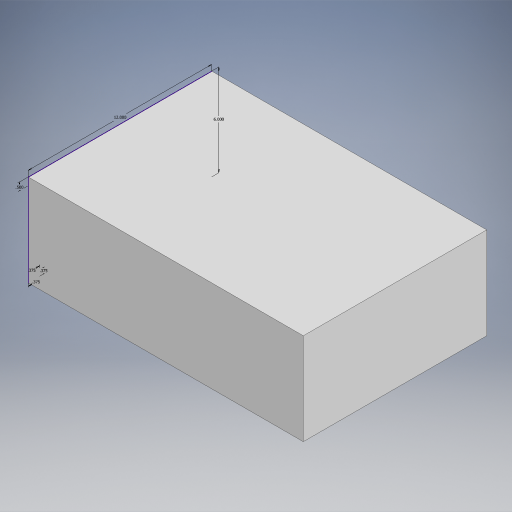
# Autodesk Inventor part: Typ_rect-01
Saved by Autodesk Inventor 2023 (Build 270158000, 158)
## iProperties
RuleStatus: InUse
Created: 2022-10-23
Part Number: Typ_rect-01
Material: Generic
Document SubType Name: Modeling
Designer: awelt
Mass: 21237.6 g
Surface Area: 5109.67 cm^2
Volume: 21237.6 cm^3
Density: 1 g/cm^3
Appearance: Default
AfterAnyParamChange0: BoundingBox
AfterAnyiPropertyChange0: BoundingBox
PartBodyChanged0: BoundingBox
BoundingBL1: 6
BoundingBL2: 12
BoundingBL3: 18
BoundingCF: 0.75
Author: awelt
Autodesk Inventor part; units mm, degrees
ref_plane "YZ Plane" through (0, 0, 0) normal (1, 0, 0) x (0, 1, 0)
ref_plane "XZ Plane" through (0, 0, 0) normal (0, 1, 0) x (-1, 0, 0)
ref_plane "XY Plane" through (0, 0, 0) normal (0, 0, 1) x (1, 0, 0)
sketch "Sketch2" plane through (0, 0, 0) normal (1, 0, 0) x (0, 1, 0)
  line L0 (0, 0) -> (152.4, 0)
  line L1 (152.4, 0) -> (152.4, -304.8)
  line L2 (152.4, -304.8) -> (0, -304.8)
  line L3 (0, -304.8) -> (0, 0)
  line L4 (152.4, -304.8) -> (139.7, 0)
  line L5 (0, -9.525) -> (9.525, -9.525)
  line L6 (9.525, -9.525) -> (9.525, -19.05)
  line L7 (9.525, -19.05) -> (0, -19.05)
  line L8 (0, -19.05) -> (0, -9.525)
  point P0 (0, -19.05)
  dimension "DimC" = 152.4
  dimension "DimB" = 304.8
  dimension "wash" = 12.7
  dimension "driph" = 9.525
  dimension "dripw" = 9.525
  dimension "dripsb" = 9.525
  constraints: 18 end point, 4 parallel, 2 horizontal, 2 perpendicular, 2 point on line
  measures "DimC" distance of L1.end L2.end
  measures "DimB" distance of L0.end L1.end
  measures "wash" distance of L4.end L0.end
  measures "driph" distance of L6.end L7.end
  measures "dripw" distance between parallel lines of L5 L7
  measures "dripsb" distance from line of L0.start L5
extrude "Main" add sketch "Sketch2" along normal blind 457.2
extrude "Wash" [suppressed]
extrude "Drip" [suppressed]
body "Solid2"
